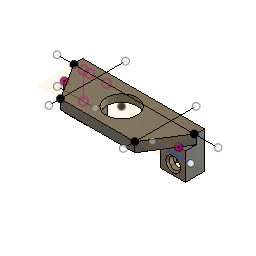
encoder-bracket (Autodesk Fusion 360 design; units mm, degrees)
Autodesk Fusion 360 part; units mm, degrees
box "BoxPrimitive1" add length 15.24 width 39.878 height 3.175 placed x (0, 0, 1) y (1, 0, 0) z (0, 1, 0) at (0, 0, 0)
sketch "Sketch3" plane through (0, 3.175, 0) normal (0, 1, 0) x (-1, 0, 0)
  line L0 (0, 15.24) -> (-39.878, 15.24)
  line L1 (-39.878, 15.24) -> (-39.878, 0)
  line L2 (-39.878, 0) -> (0, 0)
  line L3 (0, 0) -> (0, 15.24)
  circle A0 centre (-19.939, 7.3025) radius 5.08
  line L4 (5.5673, 3.175) -> (-47.7727, 3.175)
  line L5 (-7.62, -6.35) -> (-7.62, 19.05)
  line L6 (0, 3.175) -> (-7.62, 15.24)
  line L7 (-32.258, -5.08) -> (-32.258, 19.0381)
  line L8 (-32.258, 15.24) -> (-39.878, 3.175)
  dimension "d6" = 10.16
  dimension "d7" = 19.939
  dimension "d8" = 7.3025
  dimension "d15" = 3.175
  dimension "d16" = 7.62
  dimension "d17" = 7.62
  measures "d6" diameter of A0
  measures "d7" distance of L3
  measures "d15" distance of L2.end
  measures "d16" distance of L2.end
  measures "d17" distance of L2.end
hole "Hole1" at (19.939, 0, 7.3025) direction (0, 1, 0) diameter 10.16 depth 10.16 tip angle 90 counterbore diameter 12.7 counterbore depth 0.762
extrude "Extrude1" cut sketch "Sketch3" against normal blind 3.175 contours L0 L3 L6
extrude "Extrude2" cut sketch "Sketch3" against normal blind 3.175 contours L0 L1 L8
box "BoxPrimitive2" add length 9.017 width 7.62 height 6.35 placed x (0, -1, 0) y (1, 0, 0) z (0, 0, 1) at (0, 0, 0)
hole "Hole2" at (3.81, -5.842, 6.35) direction (0, 0, -1) diameter 3.81 depth 6.35 tip angle 180
box "BoxPrimitive3" add length 9.017 width 7.62 height 6.35 placed x (0, -1, 0) y (1, 0, 0) z (0, 0, 1) at (32.258, 0, 0)
hole "Hole3" at (36.068, -5.842, 6.35) direction (0, 0, -1) diameter 3.81 depth 6.35 tip angle 180
sketch "Sketch6" plane through (0, 0, 0) normal (0, 0, 1) x (1, 0, 0)
  line L0 (7.62, 0) -> (2.0053, 0)
  line L1 (0, 0) -> (0, -9.017)
sketch "Sketch7" plane through (0, 0, 6.35) normal (0, 0, 1) x (1, 0, 0)
  circle A0 centre (3.81, -5.842) radius 1.905
  line L0 (0, -9.017) -> (7.62, -9.017)
  line L1 (7.62, -9.017) -> (7.62, 0)
  line L2 (7.62, 0) -> (2.0053, 0)
  line L3 (0, 0) -> (0, -9.017)
  line L4 (-2.286, -2.667) -> (10.16, -2.667)
  line L5 (2.0053, 0) -> (0, 0)
  dimension "d40" = 6.35
  measures "d40" distance of L0
sketch "Sketch8" plane through (0, 0, 6.35) normal (0, 0, 1) x (1, 0, 0)
  circle A0 centre (36.068, -5.842) radius 1.905
  line L0 (32.258, -9.017) -> (39.878, -9.017)
  line L1 (39.878, -9.017) -> (39.878, 0)
  line L2 (37.8727, 0) -> (32.258, 0)
  line L3 (32.258, 0) -> (32.258, -9.017)
  line L4 (29.21, -2.667) -> (41.91, -2.667)
  line L5 (39.878, 0) -> (37.8727, 0)
  dimension "d43" = 6.35
  measures "d43" distance of L0
sketch "Sketch9" plane through (0, 0, 0) normal (0, -1, 0) x (1, 0, 0)
  line L0 (32.258, 6.35) -> (37.8727, 6.35)
  line L1 (37.8727, 6.35) -> (32.258, 15.24)
  line L2 (32.258, 15.24) -> (7.62, 15.24)
  line L3 (7.62, 15.24) -> (2.0053, 6.35)
  line L4 (2.0053, 6.35) -> (7.62, 6.35)
  line L5 (7.62, 6.35) -> (7.62, 0)
  line L6 (7.62, 0) -> (32.258, 0)
  line L7 (32.258, 0) -> (32.258, 6.35)
  circle A0 centre (19.939, 7.3025) radius 6.35
  line L8 (19.939, 7.3025) -> (19.939, 21.5253)
  line L9 (30.099, 20.32) -> (30.099, -2.54)
  line L10 (19.939, 7.3025) -> (43.18, 7.3025)
  line L11 (31.369, 5.3975) -> (28.829, 5.3975)
  line L12 (28.829, 5.3975) -> (28.829, 9.2075)
  line L13 (28.829, 9.2075) -> (31.369, 9.2075)
  line L14 (31.369, 9.2075) -> (31.369, 5.3975)
  line L15 (31.369, 5.3975) -> (28.829, 9.2075) construction
  line L16 (28.829, 5.3975) -> (31.369, 9.2075) construction
  dimension "d46" = 10.16
  dimension "d47" = 3.81
  dimension "d48" = 2.54
  measures "d46" distance of L8 L9
  measures "d47" distance of L11 L13
  measures "d48" distance of L12 L14
extrude "Extrude5" cut sketch "Sketch9" against normal blind 1.905 contours L9 L10 L11 L14 | L9 L10 L13 L14 | L9 L10 L11 L12 | L9 L10 L12 L13
sketch "Sketch12" plane through (0, -9.017, 0) normal (0, -1, 0) x (1, 0, 0)
  line L0 (0, 6.35) -> (0, 0)
  line L1 (0, 0) -> (7.62, 0)
  line L2 (7.62, 0) -> (7.62, 6.35)
  line L3 (7.62, 6.35) -> (0, 6.35)
  line L4 (0.635, 4.445) -> (6.985, 4.445)
  line L5 (6.985, 4.445) -> (6.985, 1.905)
  line L6 (6.985, 1.905) -> (0.635, 1.905)
  line L7 (0.635, 1.905) -> (0.635, 4.445)
  line L8 (7.62, -6.35) -> (7.62, 19.05)
  dimension "d51" = 2.54
  dimension "d52" = 6.35
  dimension "d53" = 1.905
  dimension "d61" = 0.635
  measures "d51" distance of L4 L6
  measures "d52" distance of L5 L7
  measures "d53" distance of L1 L6
  measures "d61" distance of L5 L8
extrude "Extrude6" cut sketch "Sketch12" against normal blind 6.35 contours L4 L5 L6 L7
sketch "Sketch13" plane through (0, -9.017, 0) normal (0, -1, 0) x (1, 0, 0)
  line L0 (32.258, 6.35) -> (32.258, 0)
  line L1 (32.258, 0) -> (39.878, 0)
  line L2 (39.878, 0) -> (39.878, 6.35)
  line L3 (39.878, 6.35) -> (32.258, 6.35)
  line L4 (39.243, 1.905) -> (32.893, 1.905)
  line L5 (32.893, 1.905) -> (32.893, 4.445)
  line L6 (32.893, 4.445) -> (39.243, 4.445)
  line L7 (39.243, 4.445) -> (39.243, 1.905)
  line L8 (32.258, -5.08) -> (32.258, 19.0381)
  dimension "d56" = 2.54
  dimension "d57" = 6.35
  dimension "d58" = 1.905
  dimension "d62" = 0.635
  measures "d56" distance of L4 L6
  measures "d57" distance of L5 L7
  measures "d58" distance of L1 L4
  measures "d62" distance of L5 L8
extrude "Extrude7" cut sketch "Sketch13" against normal blind 6.35 contours L4 L5 L6 L7
move_face "OffsetFaces1" offset 0.254 2 faces at (39.878, -6.0113, 3.175) (39.878, 1.0583, 2.1167)
move_face "OffsetFaces2" offset 0.254 1 faces at (32.258, -6.0113, 2.1167)
move_face "OffsetFaces3" offset 0.254 1 faces at (7.62, -6.0113, 2.1167)
move_face "OffsetFaces4" offset 0.254 1 faces at (0, -6.0113, 3.175)
chamfer "Chamfer1" distance 0.508 angle 45 4 edges at (34.2919, -6.5309, 0) (2.0339, -6.5309, 0) (34.2919, -5.1531, 6.35) (2.0339, -5.1531, 6.35)
